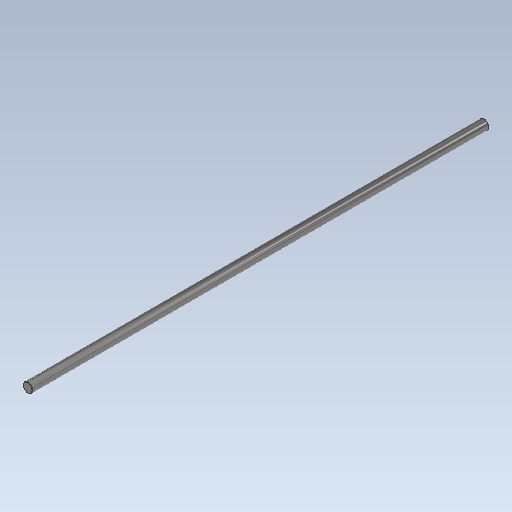
# Autodesk Inventor part: Cartesian1_12mm_Rod
Saved by Autodesk Inventor 2020 (Build 240168000, 168)
## iProperties
Created: 2020-02-29
Part Number: Cartesian1_12mm_Rod
Material: Stal, węglowa
Document SubType Name: Modeling
Designer: invin
Density: 7.85 g/cm^3
Appearance: Stal — polerowana
Mass: 500.655 g
Surface Area: 214.658 cm^2
Volume: 63.7777 cm^3
Author: invin
Autodesk Inventor part; units mm, degrees
ref_plane "YZ Plane" through (0, 0, 0) normal (1, 0, 0) x (0, 1, 0)
ref_plane "XZ Plane" through (0, 0, 0) normal (0, 1, 0) x (-1, 0, 0)
ref_plane "XY Plane" through (0, 0, 0) normal (0, 0, 1) x (1, 0, 0)
sketch "Szkic1" plane through (0, 0, 0) normal (0, 0, 1) x (1, 0, 0)
  circle A0 centre (0, 0) radius 6
  dimension "d0" = 12
  constraints: 1 centre point, 1 coincident
  measures "d0" diameter of A0
extrude "Wyciągnięcie proste1" add sketch "Szkic1" along normal blind 564
chamfer "Faza1" distance 0.5 angle 45 2 edges at (-6, 0, 564) (-6, 0, 0)
